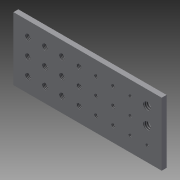
# Autodesk Inventor part: Bolt Holder
Saved by Autodesk Inventor 2013 (Build 170138000, 138)
## iProperties
Created: 2013-09-27
Part Number: Bolt Holder
Material: Generic
Document SubType Name: Modeling
Designer: grtstudent
Density: 1 g/cm^3
Author: grtstudent
Autodesk Inventor part; units mm, degrees
ref_plane "YZ Plane" through (0, 0, 0) normal (1, 0, 0) x (0, 1, 0)
ref_plane "XZ Plane" through (0, 0, 0) normal (0, 1, 0) x (-1, 0, 0)
ref_plane "XY Plane" through (0, 0, 0) normal (0, 0, 1) x (1, 0, 0)
sketch "Sketch1" plane through (0, 0, 0) normal (0, 0, 1) x (1, 0, 0)
  line L0 (0, 0) -> (96.8375, 0)
  line L1 (96.8375, 0) -> (96.8375, 41.275)
  line L2 (96.8375, 41.275) -> (0, 41.275)
  line L3 (0, 41.275) -> (0, 0)
  circle A0 centre (87.3125, 31.75) radius 7.112
  circle A1 centre (76.2, 31.75) radius 2.3241
  circle A2 centre (65.0875, 31.75) radius 3.3274
  circle A3 centre (42.8625, 31.75) radius 3.9624
  circle A4 centre (31.75, 31.75) radius 3.9624
  point P0 (9.525, 9.525)
  point P1 (9.525, 20.6375)
  point P2 (9.525, 31.75)
  point P3 (20.6375, 9.525)
  point P4 (20.6375, 20.6375)
  point P5 (20.6375, 31.75)
  point P6 (31.75, 9.525)
  point P7 (31.75, 20.6375)
  point P8 (42.8625, 9.525)
  point P9 (42.8625, 20.6375)
  point P10 (53.975, 9.525)
  point P11 (53.975, 20.6375)
  point P12 (53.975, 31.75)
  point P13 (65.0875, 9.525)
  point P14 (65.0875, 20.6375)
  point P15 (76.2, 9.525)
  point P16 (76.2, 20.6375)
  point P17 (87.3125, 9.525)
  point P18 (87.3125, 20.6375)
  dimension "d0" = 9.525
  dimension "d2" = 9.525
  dimension "d5" = 11.1125
  dimension "d8" = 11.1125
  dimension "d11" = 9.525
  dimension "d12" = 9.525
  dimension "d50" = 14.224
  dimension "d51" = 4.6482
  dimension "d52" = 6.6548
  dimension "d53" = 7.9248
  dimension "d54" = 7.9248
  constraints: 8 end point, 5 centre point, 5 coincident, 2 horizontal, 2 parallel, 1 perpendicular, 1 vertical, 23 other
  measures "d0" distance from line of L0 point (9.525, 9.525)
  measures "d2" distance from line of L3 point (9.525, 9.525)
  measures "d5" distance of point (9.525, 9.525) point (9.525, 20.638)
  measures "d8" distance of point (9.525, 9.525) point (20.637, 9.525)
  measures "d11" distance from line of L2 point (9.525, 31.75)
  measures "d12" distance from line of L1 point (87.312, 31.75)
  measures "d50" diameter of A0
  measures "d51" diameter of A1
  measures "d52" diameter of A2
  measures "d53" diameter of A3
  measures "d54" diameter of A4
extrude "Extrusion1" add sketch "Sketch1" along normal blind 3.175 contours L3 L2 L1 L0 | A0 | A1 | A2 | A3 | A4
hole "10-32" at (9.525, 9.525, 0) at (9.525, 20.6375, 0) at (9.525, 31.75, 0) at (20.6375, 9.525, 0) at (20.6375, 20.6375, 0) at (20.6375, 31.75, 0) at (31.75, 9.525, 0) at (31.75, 20.6375, 0) at (31.75, 31.75, 0) direction (0, 0, 1) diameter 3.9624 end through all thread size "10-32 UNF" class "2B" standard "ANSI Unified Screw Threads"
hole "8-32" at (42.8625, 31.75, 0) at (42.8625, 20.6375, 0) at (42.8625, 9.525, 0) direction (0, 0, 1) diameter 3.302 end through all thread size "8-32 UNC" class "2B" standard "ANSI Unified Screw Threads"
hole "6-32" at (53.975, 9.525, 0) at (53.975, 20.6375, 0) at (53.975, 31.75, 0) at (65.0875, 9.525, 0) at (65.0875, 20.6375, 0) at (65.0875, 31.75, 0) direction (0, 0, 1) diameter 2.6416 end through all thread size "6-32 UNC" class "2B" standard "ANSI Unified Screw Threads"
hole "4-40" at (76.2, 9.525, 0) at (76.2, 20.6375, 0) at (76.2, 31.75, 0) at (87.3125, 9.525, 0) direction (0, 0, 1) diameter 2.159 end through all
hole "1/4-20" at (87.3125, 20.6375, 0) at (87.3125, 31.75, 0) direction (0, 0, 1) diameter 4.9784 end through all thread size "1/4-20 UNC" class "2B" standard "ANSI Unified Screw Threads"
equation "\"d2\" = d0"
equation "\"d5\" = d8"
equation "\"d11\" = d2"
equation "\"d12\" = d0"
body "Solid1"
